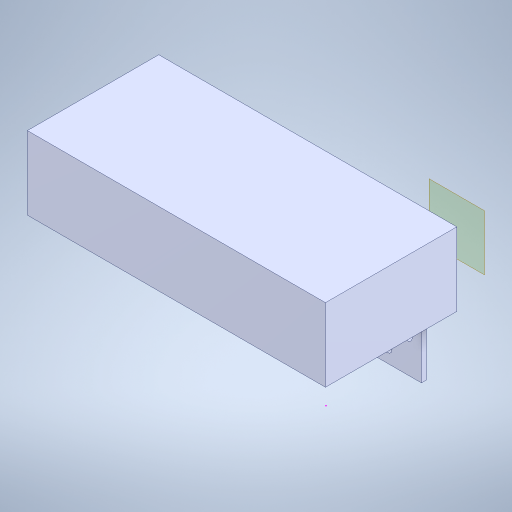
# Autodesk Inventor part: batteryMount
Saved by Autodesk Inventor 2024.2 (Build 282272000, 272)
## iProperties
Created: 2017-01-16
Part Number: batteryMount
Material: Generic
Description: STEP AP214
Document SubType Name: Modeling
Designer: student
Density: 1 g/cm^3
Appearance: Default
Sending System: SolidWorks 2016
Preprocessor: SwSTEP 2.0
Title: 39057 TETRIX 12V 3000mAH Battery Pack Assembly.STEP
Revision Number: ANY
Autodesk Inventor part; units mm, degrees
ref_plane "YZ Plane" through (0, 0, 0) normal (1, 0, 0) x (0, 1, 0)
ref_plane "XZ Plane" through (0, 0, 0) normal (0, 1, 0) x (-1, 0, 0)
ref_plane "XY Plane" through (0, 0, 0) normal (0, 0, 1) x (1, 0, 0)
ref_plane "Work Plane7" through (-37.2167, 31.2213, -6.3329) normal (0, 1, 0) x (1, 0, 0)
sketch "Sketch1" plane through (-37.2167, 31.2213, -6.3329) normal (0, 1, 0) x (1, 0, 0)
  arc A0 (-58.7242, 8.25) -> (-74.6429, -6.8045) centre (-66, 0) ccw projected
  line L0 (-77, 0) -> (-77, -32.6485)
  arc A1 (-74.6429, -15.1955) -> (-58.7242, -30.25) centre (-66, -22) ccw projected
  line L1 (-66, -33) -> (-77, -33)
  line L2 (-77, -32.6485) -> (-77, -33)
  line L3 (-77, 0) -> (-77, 11)
  arc A2 (30, -7.5498) -> (14.7242, 8.25) centre (22, 0) ccw projected
  line L4 (22, 11) -> (-77, 11)
  line L5 (-66, -33) -> (33, -33)
  arc A3 (14.7242, -30.25) -> (30, -14.4502) centre (22, -22) ccw projected
  line L6 (33, -22) -> (33, -33)
  line L7 (33, -22) -> (33, 11)
  line L8 (22, 11) -> (33, 11)
  line L9 (-79, -32.6485) -> (-79, 0)
  line L10 (-79, 0) -> (-79, 13)
  line L11 (-79, 13) -> (22, 13)
  line L12 (22, 13) -> (35, 13)
  line L13 (35, 13) -> (35, -22)
  line L14 (35, -22) -> (35, -35)
  line L15 (35, -35) -> (-66, -35)
  line L16 (-66, -35) -> (-79, -35)
  line L17 (-79, -35) -> (-79, -32.6485)
  line L18 (-81, 15) -> (-81, 0)
  line L19 (-81, 0) -> (-81, -32.6485)
  line L20 (-81, -32.6485) -> (-81, -37)
  line L21 (-81, -37) -> (-66, -37)
  line L22 (-66, -37) -> (37, -37)
  line L23 (37, -37) -> (37, -22)
  line L24 (37, -22) -> (37, 15)
  line L25 (37, 15) -> (22, 15)
  line L26 (22, 15) -> (-81, 15)
  point P0 (37.2167, -6.3329)
  dimension "d0" = 2
  dimension "d1" = 4
  constraints: 54 end point, 9 perpendicular, 5 tangent, 4 point on circle, 3 horizontal, 3 vertical, 16 other
  measures "d0" distance between parallel lines of L0 L9
  measures "d1" distance between parallel lines of L4 L26
extrude "Extrusion1" add sketch "Sketch1" against normal blind 25 contours L26 L25 L24 L23 L22 L21 L20 L19 L18
extrude "Extrusion2" add sketch "Sketch1" along normal blind 4 contours L4 A2 L7 A3 L5 A1 L0 A0 | A0 L3 L4 | L8 L7 A2 | A1 L1 L2 L0 | L6 L5 A3 | L9 L10 L11 L12 L13 L14 L15 L16 L17 | L26 L25 L24 L23 L22 L21 L20 L19 L18
sketch "Sketch3" plane through (-118.2167, 6.2213, 30.6671) normal (0, 0, 1) x (1, 0, 0)
  point P0 (118.2167, -6.2213)
sketch "Sketch4" plane through (-118.2167, 6.2213, 30.6671) normal (0, 0, 1) x (1, 0, 0)
  point P0 (118.2167, -6.2213)
ref_plane "Work Plane2" through (-37.2167, 6.2213, -6.3329) normal (0, -1, 0) x (1, 0, 0)
sketch "Sketch5" plane through (-37.2167, 6.2213, -6.3329) normal (0, -1, 0) x (1, 0, 0)
  line L0 (35, -13) -> (-79, -13) projected
  line L1 (35, -13) -> (35, -15)
  line L2 (-81, -15) -> (37, -15) projected
  line L3 (-79, 35) -> (-79, -13) projected
  line L4 (-79, -13) -> (-79, -15)
  line L5 (-79, -15) -> (35, -15)
  line L6 (35, -15) -> (25, -15)
  line L7 (25, -15) -> (25, -13)
  line L8 (25, -13) -> (-2, -13)
  line L9 (-2, -13) -> (-2, -15)
  line L10 (25, -15) -> (-2, -15)
  line L11 (-79, -15) -> (-69, -15)
  line L12 (-69, -15) -> (-69, -13)
  line L13 (-69, -13) -> (-42, -13)
  line L14 (-42, -13) -> (-42, -15)
  line L15 (-69, -15) -> (-42, -15)
  point P0 (37.2167, 6.3329)
  point P1 (-2, -15)
  point P2 (25, -15)
  point P3 (-42, -15)
  point P4 (-69, -15)
  dimension "d30" = 10
  dimension "d31" = 27
  dimension "d32" = 10
  dimension "d33" = 27
  constraints: 26 end point, 9 point on line, 5 perpendicular, 2 collinear, 2 vertical
  measures "d30" distance of L1.end L6.end
  measures "d31" distance of L7.end L8.end
  measures "d32" distance of L4.end L11.end
  measures "d33" distance of L12.end L13.end
extrude "Extrusion3" add sketch "Sketch5" along normal blind 29.5 contours L7 L2 L9 L0 | L14 L2 L12 L0
ref_plane "Work Plane3" through (-0.2167, 35.2213, -21.3329) normal (0, 0, -1) x (-1, 0, 0)
sketch "Sketch6" plane through (-0.2167, 35.2213, -21.3329) normal (0, 0, -1) x (-1, 0, 0)
  line L0 (106, -58.5) -> (79, -58.5) projected
  line L1 (106, -58.5) -> (92.5, -58.5)
  line L2 (92.5, -58.5) -> (92.5, -53)
  circle A0 centre (92.5, -53) radius 1.85
  line L3 (92.5, -53) -> (92.5, -45)
  circle A1 centre (92.5, -45) radius 4
  line L4 (92.5, -45) -> (92.5, -37)
  circle A2 centre (92.5, -37) radius 1.85
  line L5 (92.5, -45) -> (84.5, -45)
  line L6 (93.7399, -45) -> (90.2601, -45) projected
  line L7 (84.5, -45) -> (100.5, -45)
  circle A3 centre (100.5, -45) radius 1.85
  circle A4 centre (84.5, -45) radius 1.85
  line L8 (79, -29) -> (39, -29) projected
  line L9 (79, -29) -> (59, -29)
  line L10 (59, -29) -> (59, -58.5)
  circle A5 centre (25.5, -53) radius 1.85
  circle A6 centre (25.5, -45) radius 4
  circle A7 centre (25.5, -37) radius 1.85
  circle A8 centre (17.5, -45) radius 1.85
  circle A9 centre (33.5, -45) radius 1.85
  point P0 (-0.2167, -35.2213)
  dimension "d36" = 5.5
  dimension "d37" = 3.7
  dimension "d38" = 8
  dimension "d39" = 8
  dimension "d40" = 8
  dimension "d41" = 3.7
  dimension "d42" = 8
  dimension "d43" = 16
  dimension "d44" = 3.7
  dimension "d45" = 3.7
  dimension "d46" = 20
  constraints: 16 end point, 10 centre point, 6 coincident, 6 symmetric about line, 2 midpoint, 2 perpendicular, 2 vertical, 1 collinear, 1 point on line, 5 other
  measures "d36" distance of L1.end L2.end
  measures "d37" diameter of A0
  measures "d38" distance of L3.start L3.end
  measures "d39" diameter of A1
  measures "d40" distance of L4.start L4.end
  measures "d41" diameter of A2
  measures "d42" distance of L4.start L5.end
  measures "d43" distance of L5.end L7.end
  measures "d44" diameter of A3
  measures "d45" diameter of A4
  measures "d46" distance of L8.start L9.end
extrude "Extrusion4" cut sketch "Sketch6" against normal blind 2.25
body "Solid1"
